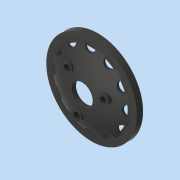
# Autodesk Inventor part: SpurGearLarge
Saved by Autodesk Inventor 2017 (Build 210142000, 142)
## iProperties
Created: 2016-11-06
Part Number: SpurGearLarge
Material: ABS Plastic
Document SubType Name: Modeling
Designer: techn
Density: 1.06 g/cm^3
Appearance: Smooth - Black
Author: techn
Autodesk Inventor part; units mm, degrees
ref_plane "YZ Plane" through (0, 0, 0) normal (1, 0, 0) x (0, 1, 0)
ref_plane "XZ Plane" through (0, 0, 0) normal (0, 1, 0) x (-1, 0, 0)
ref_plane "XY Plane" through (0, 0, 0) normal (0, 0, 1) x (1, 0, 0)
sketch "Sketch5" plane through (0, 0, 0) normal (0, 0, 1) x (1, 0, 0)
  circle A0 centre (0, 0) radius 22.86
  circle A1 centre (0, 0) radius 18.415
  dimension "d23" = 45.72
  dimension "d24" = 36.83
  constraints: 2 centre point, 2 coincident
  measures "d23" diameter of A0
  measures "d24" diameter of A1
extrude "Extrusion5" add sketch "Sketch5" along normal blind 3.175
sketch "Sketch6" plane through (0, 0, 0) normal (1, 0, 0) x (0, 1, 0)
  line L0 (22.86, 3.175) -> (-22.86, 3.175) projected
  line L1 (-22.86, 0) -> (22.86, 0) projected
  line L2 (22.86, 3.175) -> (-22.86, 3.175) projected
  line L3 (0, 3.175) -> (5.461, 3.175)
  line L4 (5.461, 3.175) -> (5.461, 7.9375)
  line L5 (22.86, 3.175) -> (19.685, 3.175)
  arc A0 (19.685, 3.175) -> (5.461, 7.9375) centre (0.0858, -31.7388) ccw
  line L6 (0, 3.175) -> (0, 13.9666)
  line L7 (-18.415, 3.175) -> (18.415, 3.175) projected
  line L8 (19.685, 3.175) -> (18.415, 3.175)
  arc A1 (18.415, 3.175) -> (5.461, 5.715) centre (1.4326, -49.1328) ccw
  point P0 (0, 0)
  dimension "d27" = 5.461
  dimension "d28" = 4.7625
  dimension "d29" = 3.175
  dimension "d36" = 2.54
  constraints: 10 end point, 4 point on circle, 3 point on line, 2 centre point, 1 horizontal, 1 midpoint, 1 perpendicular, 1 vertical
  measures "d27" distance of L3.start L3.end
  measures "d28" distance of L3.end L4.end
  measures "d29" distance of L0.start L5.end
  measures "d36" distance of L3.end A1.end
revolve "Revolution3" add sketch "Sketch6" angle 360 about axis through (0, 0, 3.175) along (0, 0, 1) contours L0 A1 L4 A0
sketch "Sketch8" plane through (0, 0, 3.175) normal (0, 0, 1) x (1, 0, 0)
  circle A0 centre (0, 0) radius 19.685 projected
  circle A1 centre (0, 19.685) radius 2.8575
  circle A2 centre (-9.8425, 17.0477) radius 2.8575
  circle A3 centre (-17.0477, 9.8425) radius 2.8575
  circle A4 centre (-19.685, 0) radius 2.8575
  circle A5 centre (-17.0477, -9.8425) radius 2.8575
  circle A6 centre (-9.8425, -17.0477) radius 2.8575
  circle A7 centre (0, -19.685) radius 2.8575
  circle A8 centre (9.8425, -17.0477) radius 2.8575
  circle A9 centre (17.0477, -9.8425) radius 2.8575
  circle A10 centre (19.685, 0) radius 2.8575
  circle A11 centre (17.0477, 9.8425) radius 2.8575
  circle A12 centre (9.8425, 17.0477) radius 2.8575
  dimension "d38" = 5.715
  dimension "d41" = 360
  constraints: 12 centre point, 1 vertical alignment, 26 other
  measures "d38" diameter of A1
extrude "Extrusion6" cut sketch "Sketch8" along normal blind 3.175 contours A0 A10 | A0 A10 | A11 A0 | A0 A11 | A9 A0 | A0 A9 | A12 A0 | A0 A12 | A8 A0 | A0 A8 | A1 A0 | A0 A1 | A7 A0 | A0 A7 | A2 A0 | A0 A2 | A6 A0 | A0 A6 | A3 A0 | A0 A3 | A5 A0 | A0 A5 | A4 A0 | A0 A4
ref_plane "Work Plane1" through (0, 0, 7.9375) normal (0, 0, 1) x (1, 0, 0)
sketch "Sketch9" plane through (0, 0, 7.9375) normal (0, 0, 1) x (1, 0, 0)
  line L0 (0, 0) -> (12.7, 0) construction
  circle A0 centre (-7.7771, 7.7771) radius 1.5875
  circle A1 centre (-7.7771, 7.7771) radius 2.54
  circle A2 centre (-2.8466, -10.6238) radius 2.54
  circle A3 centre (-2.8466, -10.6238) radius 1.5875
  circle A4 centre (10.6238, 2.8466) radius 2.54
  circle A5 centre (10.6238, 2.8466) radius 1.5875
  dimension "d48" = 3.175
  dimension "d49" = 5.08
  dimension "d52" = 360
  dimension "d58" = 19.05
  constraints: 6 centre point, 3 coincident, 2 end point, 1 horizontal, 13 other
  measures "d48" diameter of A0
  measures "d49" diameter of A1
  measures "d58" distance of A4.centre A0.centre
extrude "Extrusion7" add sketch "Sketch9" against normal blind 2.286
extrude "Extrusion8" cut sketch "Sketch9" against normal through all contours A0 | A3 | A5
body "Solid2"
